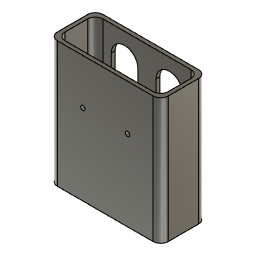
trinitron-remote-holder (Autodesk Fusion 360 design; units mm, degrees)
Autodesk Fusion 360 part; units mm, degrees
sketch "top" plane through (0, 0, 0) normal (0, 0, 1) x (1, 0, 0)
  line L0 (0, 0) -> (68, 0)
  line L1 (68, 0) -> (68, -25)
  line L2 (68, -25) -> (0, -25)
  line L3 (0, -25) -> (0, 0)
  line L4 (70.5, -27.5) -> (-2.5, -27.5)
  line L5 (-2.5, -27.5) -> (-2.5, 2.5)
  line L6 (-2.5, 2.5) -> (70.5, 2.5)
  line L7 (70.5, 2.5) -> (70.5, -27.5)
  dimension "d1" = 68
  dimension "d2" = 25
  dimension "d3" = -2.5
  constraint horizontal L0
  constraint vertical L1
  constraint horizontal L2
  constraint vertical L3
  constraint coincident L0.start L3.end
  measures "d1" distance of L0.start L0.end
  measures "d2" distance of L0.start L2.end
extrude "Extrude1" add sketch "top" along normal blind 3 contours L0 L1 L2 L3 | L4 L5 L6 L7
extrude "Extrude2" add sketch "top" along normal blind 80 from surface at 3
fillet "Fillet1" radius 5 8 edges at (-2.5, -27.5, 41.5) (70.5, -27.5, 41.5) (70.5, 2.5, 41.5) (0, 0, 43) (0, -25, 43) (68, -25, 43) (68, 0, 43) (-2.5, 2.5, 41.5)
sketch "side" plane through (0, 2.5, 0) normal (0, 1, 0) x (-1, 0, 0)
  line L0 (-2.5, 0) -> (-2.5, 83)
  line L1 (-2.5, 83) -> (-65.5, 83)
  line L2 (-65.5, 83) -> (-65.5, 0)
  line L3 (-65.5, 0) -> (-2.5, 0)
  line L4 (-65.5, 0) -> (-65.5, 83)
  line L5 (-2.5, 83) -> (-2.5, 0)
  line L6 (-65.5, 83) -> (-2.5, 83)
  line L7 (-2.5, 0) -> (-65.5, 0)
  line L8 (-34, 83) -> (-34, 0) construction
  line L9 (-57.5, 66.25) -> (-57.5, 16.75)
  arc A0 (-57.5, 16.75) -> (-40, 16.75) centre (-48.75, 16.75) ccw
  line L10 (-40, 16.75) -> (-40, 66.25)
  arc A1 (-40, 66.25) -> (-57.5, 66.25) centre (-48.75, 66.25) ccw
  line L11 (-48.75, 66.25) -> (-48.75, 16.75) construction
  arc A2 (-10.5, 66.25) -> (-28, 66.25) centre (-19.25, 66.25) ccw
  line L12 (-10.5, 66.25) -> (-10.5, 16.75)
  arc A3 (-28, 16.75) -> (-10.5, 16.75) centre (-19.25, 16.75) ccw
  line L13 (-28, 16.75) -> (-28, 66.25)
  circle A4 centre (-48.75, 53) radius 1.5
  circle A5 centre (-19.25, 53) radius 1.5
  dimension "d11" = 8
  dimension "d12" = 6
  dimension "d13" = 8
  dimension "d14" = 8
  dimension "d17" = 3
  dimension "d18" = 30
  constraint midpoint L6 L8.start
  constraint midpoint L7 L8.end
  constraint tangent L9 A0
  constraint tangent A0 L10
  constraint parallel L9 L10
  constraint tangent L10 A1
  constraint tangent L9 A1
  constraint vertical L11
  constraint symmetric L8 L9.start A2.start
  constraint symmetric L8 L9.end L12.end
  constraint symmetric L8 A0.end A3.start
  constraint symmetric L8 L10.end A2.end
  constraint symmetric L8 A0 A3
  constraint symmetric L8 A1 A2
  constraint coincident L11 A4.centre
  constraint symmetric L8 A4 A5
  measures "d11" distance of L4 L9
  measures "d12" distance of L8 L10
  measures "d13" distance of L6 A1
  measures "d14" distance of L3 A0
  measures "d17" diameter of A4
  measures "d18" distance of L1 A4.centre
extrude "Extrude3" cut sketch "side" against normal up to surface (2.5 mm away) contours L9 A0 L10 A1 | A2 L12 A3 L13 | A4 | A5
extrude "Extrude4" cut sketch "side" against normal up to surface (2.5 mm away) from surface at -27.5 contours A4 | A5
named bodies: "trinitron-remote-holder"
